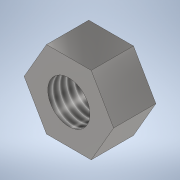
# Autodesk Inventor part: tuercaM3
Saved by Autodesk Inventor 2021.5 (Build 255421000, 421)
## iProperties
Created: 2024-11-29
Part Number: tuercaM3
Material: Acero inoxidable
Document SubType Name: Modeling
Designer: Joho_
Mass: 0.45892 g
Surface Area: 1.23668 cm^2
Volume: 0.0573649 cm^3
Density: 8 g/cm^3
Appearance: Semipulido
Author: Joho_
Autodesk Inventor part; units mm, degrees
ref_plane "YZ Plane" through (0, 0, 0) normal (1, 0, 0) x (0, 1, 0)
ref_plane "XZ Plane" through (0, 0, 0) normal (0, 1, 0) x (-1, 0, 0)
ref_plane "XY Plane" through (0, 0, 0) normal (0, 0, 1) x (1, 0, 0)
sketch "Boceto1" plane through (0, 0, 0) normal (0, 0, 1) x (1, 0, 0)
  circle A0 centre (0, 0) radius 1.5
  line L0 (0, 0) -> (3.175, 0)
  line L1 (3.175, 0) -> (1.5875, -2.7496)
  line L2 (1.5875, -2.7496) -> (-1.5875, -2.7496)
  line L3 (-1.5875, -2.7496) -> (-3.175, 0)
  line L4 (-3.175, 0) -> (-1.5875, 2.7496)
  line L5 (-1.5875, 2.7496) -> (1.5875, 2.7496)
  line L6 (1.5875, 2.7496) -> (3.175, 0)
  dimension "d0" = 3
  dimension "d1" = 3.175
  constraints: 14 end point, 2 coincident, 1 centre point, 1 horizontal, 13 other
  measures "d0" diameter of A0
  measures "d1" distance of L0.start L0.end
extrude "Extrusión1" add sketch "Boceto1" along normal mid plane 3
thread "Rosca1" size "M3x0.5" class "6H" standard "ANSI Metric M Profile" full length
